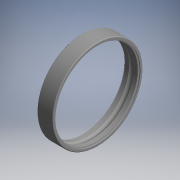
# Autodesk Inventor part: SKF_W 61703-2RS1_PART2
Saved by Autodesk Inventor 2017.3 (Build 213256000, 256)
## iProperties
Part Number: SKF_W 61703-2RS1_PART2
Material: Generic
Catalog Web Link: www.cadenas.de
Description: -Deep groove ball bearings
Vendor: SKF
Document SubType Name: Modeling
Designer: partserver
Manufacturer: SKF
Mass: 4 g
Surface Area: 6.97542 cm^2
Volume: 0.233551 cm^3
Density: 1 g/cm^3
Appearance: PSOLRGB-175-175-175
Category: PARTsolutions
Company: SKF
Title: SKF_W 61703-2RS1_PART2
Author: Cadenas PARTsolutions
Comments: Deep groove ball bearings
PSOL_IDENT_0: {$CADENAS_DATA\23d-libs\skf\bearings_units_and_housings\ball_bearings\deep_groove_ball_bearings\bb1_
PSOL_IDENT_1: 001_101.prj},211 {VTYP=3D},{NB=SKF_W 61703-2RS1_PART2},{LINA=SKF_W 61703-2RS1_PART2},{NN=BB1_001_101
PSOL_IDENT_2: _PART2},{NOPRJ=TRUE},{DATE=03.06.2022 09:06:52},{GEOMDATE=31.05.2022 11:14:58},{VERSION=},{LINEID=17
PSOL_IDENT_3: 110},{WBVAR=},{WBNUMERIC=}  {NB=SKF_W 61703-2RS1_PART2},{LINA=SKF_W 61703-2RS1_PART2},{KT=DUMMY},{DE
PSOL_IDENT_4: SIGNATION=W 61703-2RS1},{R12=0.20},{DD=17.000},{D=23.000},{B=4.000},{C=},{CX=},{CXX=},{CA=0.000},{XX
PSOL_IDENT_5: VARIANT=},{XXDESIGN=Single row stainless steel},{XXSEALING=Contact seal on both sides},{DESIGN=dgbbw
PSOL_IDENT_6: 2rs},{DESIGNIR=dgbbw2rs},{VARIANT=},{DD1=18.86},{DD2=18.86},{DD2X=},{DD2A=18.86},{D1=21.10},{D1X=0.0
PSOL_IDENT_7: 0},{D2=21.67},{D2A=21.67},{D3=},{D3X=},{D3A=0.000},{D4=},{HH=0.000},{BB=0.000},{BBX=},{BBA=0.000},{F
PSOL_IDENT_8: F=},{R0MAX=0.000},{R0=0.000},{PITCH=20.00},{DW=1.588},{DDAMIN=18.500},{DDAMAX=18.500},{DDBMIN=0.000}
PSOL_IDENT_9: ,{DDBMAX=0.000},{DBMIN=0.000},{DAMAX=22.000},{BBAMIN=0.000},{CAMAX=0.000},{RAMAX=0.200},{LOAD1=0.559
PSOL_IDENT_10: },{LOAD2=0.340},{LOAD3=0.015},{SPEED1=0},{SPEED2=17000},{KR=0.015},{F0=8.500},{Z=16},{II=1},{MASS=0.
PSOL_IDENT_11: 004},{BEARING=W 61703-2RS1},{RING=},{HELP=0.950},{HELP2=0.665},{DD1ALG=9.430},{YALG=9.430},{PITCH1=2
PSOL_IDENT_12: 0.000},{DW1=1.588},{YALG1=10.550},{HALG1=0.950},{SH=9.430},{CU=0.482},{HALG=0.93},{B1=0},{SHIELDHELP=
PSOL_IDENT_13: 2},{D4A=0.000},{FFA=0.000},{RS1=},{HELP3=0}
NB: SKF_W 61703-2RS1_PART2
NT: Deep groove ball bearings
NBSYN: SKF_$DESIGNATION._PART2
LINA: SKF_W 61703-2RS1_PART2
CATALOG: SKF
DESIGNATION: W 61703-2RS1
R12: 0.2
DD: 17
D: 23
B: 4
XXDESIGN: Single row stainless steel
XXSEALING: Contact seal on both sides
DD2: 18.86
D2: 21.67
LOAD1: 0.559
LOAD2: 0.34
LOAD3: 0.015
SPEED1: 0
SPEED2: 17000
BEARING: W 61703-2RS1
SUPPLIER: SKF
ARTICLENO: SKF_W 61703-2RS1_PART2
BOMINFO: SKF_W 61703-2RS1_PART2
CREATOR: CADENAS GmbH
Autodesk Inventor part; units mm, degrees
ref_plane "YZ Plane" through (0, 0, 0) normal (1, 0, 0) x (0, 1, 0)
ref_plane "XZ Plane" through (0, 0, 0) normal (0, 1, 0) x (-1, 0, 0)
ref_plane "XY Plane" through (0, 0, 0) normal (0, 0, 1) x (1, 0, 0)
sketch "Sketch_16" plane through (0, 0, 0) normal (0, 0, 1) x (1, 0, 0)
  line L0 (50, 0) -> (-50, 0)
  line L1 (0, 10.835) -> (0.06, 10.835)
  arc A0 (0.3, 10.835) -> (0.06, 10.835) centre (0.18, 10.835) ccw
  line L2 (0.3, 10.835) -> (0.3503, 10.55)
  line L3 (0.3503, 10.55) -> (1.4273, 10.55)
  arc A1 (2.5727, 10.55) -> (1.4273, 10.55) centre (2, 10) ccw
  line L4 (2.5727, 10.55) -> (3.6497, 10.55)
  line L5 (3.6497, 10.55) -> (3.7, 10.835)
  arc A2 (3.94, 10.835) -> (3.7, 10.835) centre (3.82, 10.835) ccw
  line L6 (3.94, 10.835) -> (4, 10.835)
  line L7 (4, 10.835) -> (4, 11.3)
  arc A3 (4, 11.3) -> (3.8, 11.5) centre (3.8, 11.3) ccw
  line L8 (3.8, 11.5) -> (0.2, 11.5)
  arc A4 (0.2, 11.5) -> (0, 11.3) centre (0.2, 11.3) ccw
  line L9 (0, 11.3) -> (0, 10.835)
  constraints: 20 end point, 10 point on circle, 5 centre point
revolve "Revolution1" add sketch "Sketch_16" angle 360 about axis through (50, 0, 0) along (1, 0, 0)
body "Solid1"
